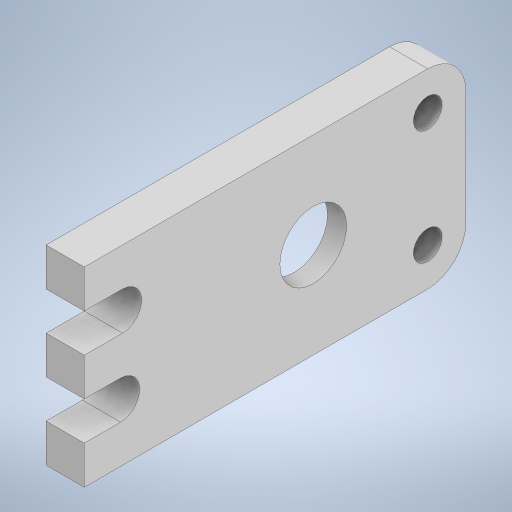
# Autodesk Inventor part: Wkp 01.03.1
Saved by Autodesk Inventor 2023 (Build 270158000, 158)
## iProperties
Created: 2023-03-01
Part Number: Wkp 01.03.1
Material: Generic
Document SubType Name: Modeling
Designer: accam
Density: 1 g/cm^3
Appearance: Default
Author: accam
Autodesk Inventor part; units mm, degrees
ref_plane "YZ Plane" through (0, 0, 0) normal (1, 0, 0) x (0, 1, 0)
ref_plane "XZ Plane" through (0, 0, 0) normal (0, 1, 0) x (-1, 0, 0)
ref_plane "XY Plane" through (0, 0, 0) normal (0, 0, 1) x (1, 0, 0)
sketch "Sketch1" plane through (0, 0, 0) normal (1, 0, 0) x (0, 1, 0)
  line L0 (0, 0) -> (10.3831, 0)
  line L1 (0, 0) -> (12.9478, 0)
  line L2 (0, 0) -> (100, 0)
  line L3 (100, 0) -> (100, -180)
  line L4 (80, -200) -> (20, -200)
  line L5 (0, -180) -> (0, 0)
  line L6 (20.0847, 0) -> (40.0847, 0)
  line L7 (60, 0) -> (80, 0)
  line L8 (80, 0) -> (80, -20)
  line L9 (70, -30) -> (70, -30)
  line L10 (60, -20) -> (60, 0)
  line L11 (40.0847, 0) -> (40.0847, -19)
  line L12 (30.0847, -29) -> (30.0847, -29)
  line L13 (0, 0) -> (0, -30)
  line L14 (20.0847, -19) -> (20.0847, 0)
  arc A0 (80, -200) -> (100, -180) centre (80, -180) ccw
  arc A1 (0, -180) -> (20, -200) centre (20, -180) ccw
  arc A2 (30.0847, -29) -> (40.0847, -19) centre (30.0847, -19) ccw
  arc A3 (20.0847, -19) -> (30.0847, -29) centre (30.0847, -19) ccw
  arc A4 (60, -20) -> (70, -30) centre (70, -20) ccw
  arc A5 (70, -30) -> (80, -20) centre (70, -20) ccw
  circle A6 centre (80, -180) radius 7.5
  circle A7 centre (20, -180) radius 7.5
  circle A8 centre (50, -120) radius 17.5
  circle A9 centre (50, -120) radius 32.5
  point P0 (100, -200)
  point P1 (0, -200)
  dimension "d0" = 100
  dimension "d1" = 200
  dimension "d10" = 20
  dimension "d16" = 20
  dimension "d23" = 15
  dimension "d24" = 35
  dimension "d25" = 65
  dimension "d26" = 50
  dimension "d31" = 80
  constraints: 30 end point, 12 point on circle, 12 tangent, 10 centre point, 7 point on line, 5 horizontal, 4 parallel, 3 perpendicular, 2 coincident, 1 vertical
  measures "d0" distance of point (100, -200) point (0, -200)
  measures "d1" distance of L2.end point (100, -200)
  measures "d10" radius of A0
  measures "d16" radius of A1
  measures "d23" diameter of A7
  measures "d24" diameter of A8
  measures "d25" diameter of A9
  measures "d26" distance from line of A9.centre L5
  measures "d31" distance from line of L4 A8.centre
extrude "Extrusion1" add sketch "Sketch1" along normal blind 20 contours L0 L1 L2 L14 A3 A2 L11 L10 A4 A5 L8 L3 A0 L4 A1 L5 | A9
extrude "Extrusion2" cut sketch "Sketch1" along normal blind 10 contours A8 | A9
body "Solid1"
